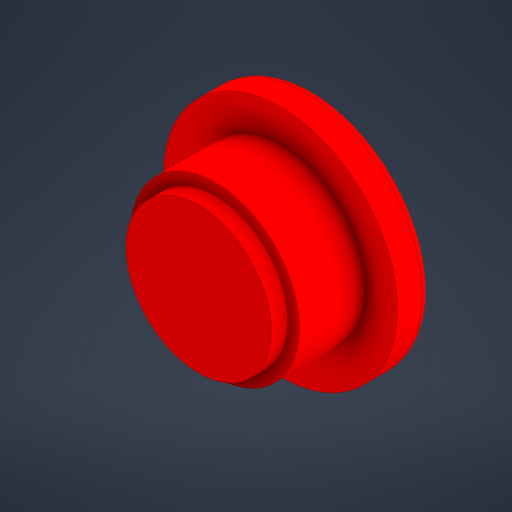
# Autodesk Inventor part: SM1 Removal Tool
Saved by Autodesk Inventor 2023.4 (Build 274418000, 418)
## iProperties
Created: 2024-07-23
Part Number: SM1 Removal Tool
Material: Generic
Document SubType Name: Modeling
Designer: xSibe
Density: 1 g/cm^3
Appearance: Plastic Red
Author: xSibe
Autodesk Inventor part; units mm, degrees
ref_plane "YZ Plane" through (0, 0, 0) normal (1, 0, 0) x (0, 1, 0)
ref_plane "XZ Plane" through (0, 0, 0) normal (0, 1, 0) x (-1, 0, 0)
ref_plane "XY Plane" through (0, 0, 0) normal (0, 0, 1) x (1, 0, 0)
sketch "Sketch1" plane through (0, 0, 0) normal (0, 0, 1) x (1, 0, 0)
  circle A0 centre (0, 0) radius 11.125
  circle A1 centre (0, 0) radius 12.875
  circle A2 centre (0, 0) radius 17.875
  dimension "d0" = 22.25
  dimension "d1" = 25.75
  dimension "d2" = 5
  constraints: 3 centre point, 2 coincident
  measures "d0" diameter of A0
  measures "d1" diameter of A1
  measures "d2" radial gap between concentric circles of A1 A2
extrude "Extrusion1" add sketch "Sketch1" along normal blind 5 contours A0 | A1 | A2
extrude "Extrusion2" add sketch "Sketch1" along normal blind 10 from surface at 5 contours A0 | A1
extrude "Extrusion3" add sketch "Sketch1" along normal blind 2.5 from surface at 15 contours A0
fillet "Fillet1" radius 1.25 1 edges at (-17.875, 0, 0)
sketch "Sketch2" plane through (0, 0, 0) normal (0, 0, -1) x (-1, 0, 0)
  line L0 (-12.5, -12.5) -> (12.5, -12.5)
  line L1 (12.5, -12.5) -> (12.5, 12.5)
  line L2 (12.5, 12.5) -> (-12.5, 12.5)
  line L3 (-12.5, 12.5) -> (-12.5, -12.5)
  line L4 (-12.5, -12.5) -> (12.5, 12.5) construction
  line L5 (12.5, -12.5) -> (-12.5, 12.5) construction
  line L6 (-12.5, 12.5) -> (12.5, 12.5) construction
  line L7 (12.5, 12.5) -> (12.5, -12.5) construction
  line L8 (12.5, -12.5) -> (-12.5, -12.5) construction
  line L9 (-12.5, -12.5) -> (-12.5, 12.5) construction
  line L10 (8.9708, -10) -> (5.5186, -10)
  line L11 (5.5186, -10) -> (-0.8023, -2.0421)
  line L12 (-0.8023, -2.0421) -> (-3.8493, -2.0421)
  line L13 (-3.8493, -2.0421) -> (-3.8493, -10)
  line L14 (-3.8493, -10) -> (-6.5073, -10)
  line L15 (-6.5073, -10) -> (-6.5073, 10)
  line L16 (-6.5073, 10) -> (-1.3533, 10)
  spline S0 degree 2 poles (-1.3533, 10) (0.3647, 10) (2.6823, 9.6272) (3.7358, 8.9465) knots 0 0 0 1 2 2 2
  spline S1 degree 2 poles (3.7358, 8.9465) (4.7893, 8.2658) (6.0049, 6.1426) (6.0049, 4.5705) knots 0 0 0 1 2 2 2
  spline S2 degree 2 poles (6.0049, 4.5705) (6.0049, 2.3825) (3.7682, -0.5835) (1.8558, -1.2966) knots 0 0 0 1 2 2 2
  line L17 (1.8558, -1.2966) -> (8.9708, -10)
  spline S3 degree 2 poles (3.2334, 4.3598) (3.2334, 5.235) (2.6175, 6.5802) (1.9692, 7.0178) knots 0 0 0 1 2 2 2
  spline S4 degree 2 poles (1.9692, 7.0178) (1.4019, 7.3906) (-0.1053, 7.6985) (-1.2075, 7.6985) knots 0 0 0 1 2 2 2
  line L18 (-1.2075, 7.6985) -> (-3.8493, 7.6985)
  line L19 (-3.8493, 7.6985) -> (-3.8493, 0.1783)
  line L20 (-3.8493, 0.1783) -> (-1.5154, 0.1783)
  spline S5 degree 2 poles (-1.5154, 0.1783) (-0.3647, 0.1783) (1.4668, 0.5835) (2.0989, 1.2156) knots 0 0 0 1 2 2 2
  spline S6 degree 2 poles (2.0989, 1.2156) (2.6823, 1.7666) (3.2334, 3.3225) (3.2334, 4.3598) knots 0 0 0 1 2 2 2
  point P0 (0, 0)
  dimension "d10" = 25
  dimension "d11" = 25
  constraints: 12 end point, 2 coincident, 2 midpoint, 2 parallel, 1 horizontal, 1 perpendicular, 2 other
  measures "d10" distance of L2.end L1.end
  measures "d11" distance of L1.end L0.end
extrude "Extrusion4" cut sketch "Sketch2" against normal blind 0.25 contours L10 L11 L12 L13 L14 L15 L16 S0 S1 S2 L17
chamfer "Chamfer1" distance 0.25 angle 45 18 edges at (-7.2447, -10, 0.25) (-2.3582, -6.0211, 0.25) (2.3258, -2.0421, 0.25) (3.8493, -6.0211, 0.25) (5.1783, -10, 0.25) (6.5073, 0, 0.25) (3.9303, 10, 0.25) (-1.5235, 9.8136, 0.25) (-5.3971, 7.2042, 0.25) (-4.8865, 0.8995, 0.25) (-5.4133, -5.6483, 0.25) (-2.9579, 2.5446, 0.25) (-2.9254, 5.9076, 0.25) (-0.6483, 7.5446, 0.25) (2.5284, 7.6985, 0.25) (3.8493, 3.9384, 0.25) (2.6823, 0.1783, 0.25) (-0.5511, 0.3809, 0.25)
body "Solid1"
